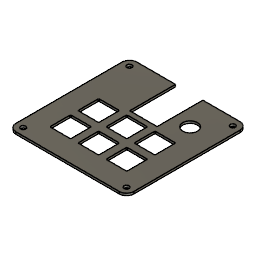
Full+Skyboard (Autodesk Fusion 360 archive; units mm, degrees)
design "TopPart"
part number: 2026-01-17-14-14-09-659
Autodesk Fusion 360 part; units mm, degrees
sketch "Sketch1" plane through (0, 0, 0) normal (0, 0, 1) x (1, 0, 0)
  line L0 (3.025, -2.525) -> (16.025, -2.525)
  line L1 (3.025, -16.525) -> (16.025, -16.525)
  line L2 (2.525, -3.025) -> (2.525, -16.025)
  line L3 (16.525, -3.025) -> (16.525, -16.025)
  arc A0 (3.025, -2.525) -> (2.525, -3.025) centre (3.025, -3.025) ccw
  arc A1 (16.525, -3.025) -> (16.025, -2.525) centre (16.025, -3.025) ccw
  arc A2 (2.525, -16.025) -> (3.025, -16.525) centre (3.025, -16.025) ccw
  arc A3 (16.025, -16.525) -> (16.525, -16.025) centre (16.025, -16.025) ccw
  line L4 (22.075, -2.525) -> (35.075, -2.525)
  line L5 (22.075, -16.525) -> (35.075, -16.525)
  line L6 (21.575, -3.025) -> (21.575, -16.025)
  line L7 (35.575, -3.025) -> (35.575, -16.025)
  arc A4 (22.075, -2.525) -> (21.575, -3.025) centre (22.075, -3.025) ccw
  arc A5 (35.575, -3.025) -> (35.075, -2.525) centre (35.075, -3.025) ccw
  arc A6 (21.575, -16.025) -> (22.075, -16.525) centre (22.075, -16.025) ccw
  arc A7 (35.075, -16.525) -> (35.575, -16.025) centre (35.075, -16.025) ccw
  line L8 (41.125, -2.525) -> (54.125, -2.525)
  line L9 (41.125, -16.525) -> (54.125, -16.525)
  line L10 (40.625, -3.025) -> (40.625, -16.025)
  line L11 (54.625, -3.025) -> (54.625, -16.025)
  arc A8 (41.125, -2.525) -> (40.625, -3.025) centre (41.125, -3.025) ccw
  arc A9 (54.625, -3.025) -> (54.125, -2.525) centre (54.125, -3.025) ccw
  arc A10 (40.625, -16.025) -> (41.125, -16.525) centre (41.125, -16.025) ccw
  arc A11 (54.125, -16.525) -> (54.625, -16.025) centre (54.125, -16.025) ccw
  line L12 (3.025, -21.575) -> (16.025, -21.575)
  line L13 (3.025, -35.575) -> (16.025, -35.575)
  line L14 (2.525, -22.075) -> (2.525, -35.075)
  line L15 (16.525, -22.075) -> (16.525, -35.075)
  arc A12 (3.025, -21.575) -> (2.525, -22.075) centre (3.025, -22.075) ccw
  arc A13 (16.525, -22.075) -> (16.025, -21.575) centre (16.025, -22.075) ccw
  arc A14 (2.525, -35.075) -> (3.025, -35.575) centre (3.025, -35.075) ccw
  arc A15 (16.025, -35.575) -> (16.525, -35.075) centre (16.025, -35.075) ccw
  line L16 (22.075, -21.575) -> (35.075, -21.575)
  line L17 (22.075, -35.575) -> (35.075, -35.575)
  line L18 (21.575, -22.075) -> (21.575, -35.075)
  line L19 (35.575, -22.075) -> (35.575, -35.075)
  arc A16 (22.075, -21.575) -> (21.575, -22.075) centre (22.075, -22.075) ccw
  arc A17 (35.575, -22.075) -> (35.075, -21.575) centre (35.075, -22.075) ccw
  arc A18 (21.575, -35.075) -> (22.075, -35.575) centre (22.075, -35.075) ccw
  arc A19 (35.075, -35.575) -> (35.575, -35.075) centre (35.075, -35.075) ccw
  line L20 (41.125, -21.575) -> (54.125, -21.575)
  line L21 (41.125, -35.575) -> (54.125, -35.575)
  line L22 (40.625, -22.075) -> (40.625, -35.075)
  line L23 (54.625, -22.075) -> (54.625, -35.075)
  arc A20 (41.125, -21.575) -> (40.625, -22.075) centre (41.125, -22.075) ccw
  arc A21 (54.625, -22.075) -> (54.125, -21.575) centre (54.125, -22.075) ccw
  arc A22 (40.625, -35.075) -> (41.125, -35.575) centre (41.125, -35.075) ccw
  arc A23 (54.125, -35.575) -> (54.625, -35.075) centre (54.125, -35.075) ccw
  line L24 (-11.052, 31.916) -> (68.948, 31.916)
  line L25 (68.948, 31.916) -> (68.948, -50.084)
  line L26 (68.948, -50.084) -> (-11.052, -50.084)
  line L27 (-11.052, -50.084) -> (-11.052, 31.916)
  line L28 (20.198, 31.916) -> (38.698, 31.916)
  line L29 (38.698, 31.916) -> (38.698, 0.916)
  line L30 (38.698, 0.916) -> (20.198, 0.916)
  line L31 (20.198, 0.916) -> (20.198, 31.916)
  circle A24 centre (-6.052, 26.916) radius 1.7
  circle A25 centre (-6.052, -45.084) radius 1.7
  circle A26 centre (63.948, -45.084) radius 1.7
  circle A27 centre (63.948, 26.916) radius 1.7
  dimension "d1" = 80
  dimension "d2" = 82
  dimension "d4" = 13.577
  dimension "d5" = 14.509
  dimension "d6" = 18.5
  dimension "d7" = 31
  dimension "d8" = 31.25
  dimension "d9" = 3.4
  dimension "d10" = 5
  dimension "d11" = 5
  dimension "d12" = 3.4
  dimension "d13" = 5
  dimension "d14" = 5
  dimension "d15" = 3.4
  dimension "d16" = 5
  dimension "d17" = 5
  dimension "d18" = 3.4
  dimension "d19" = 5
  dimension "d20" = 5
  constraint horizontal L24
  constraint vertical L25
  constraint horizontal L26
  constraint vertical L27
  constraint horizontal L28
  constraint vertical L29
  constraint horizontal L30
  constraint vertical L31
  constraint coincident L24 L28.start
  measures "d1" distance of L24.start L24.end
  measures "d2" distance of L24.start L26.end
  measures "d4" distance of L14 L27
  measures "d5" distance of L13 L26
  measures "d6" distance of L28.start L28.end
  measures "d7" distance of L28.start L30.end
  measures "d8" distance of L27 L31
  measures "d9" diameter of A24
  measures "d10" distance of L24 A24.centre
  measures "d11" distance of L27 A24.centre
  measures "d12" diameter of A25
  measures "d13" distance of L26 A25.centre
  measures "d14" distance of L27 A25.centre
  measures "d15" diameter of A26
  measures "d16" distance of L26 A26.centre
  measures "d17" distance of L25 A26.centre
  measures "d18" diameter of A27
  measures "d19" distance of L24 A27.centre
  measures "d20" distance of L25 A27.centre
extrude "Extrude1" add sketch "Sketch1" along normal blind 1.5 contours L24 L25 L26 L27 L29 L30 L31
fillet "Fillet1" radius 5 4 edges at (-11.052, -50.084, 0.75) (-11.052, 31.916, 0.75) (68.948, -50.084, 0.75) (68.948, 31.916, 0.75)
sketch "Sketch2" plane through (0, 0, 1.5) normal (0, 0, 1) x (-1, 0, 0)
  arc A0 (-68.948, -26.916) -> (-63.948, -31.916) centre (-63.948, -26.916) ccw
  line L0 (-63.948, -31.916) -> (-38.698, -31.916)
  line L1 (-38.698, -31.916) -> (-38.698, -0.916)
  line L2 (-38.698, -0.916) -> (-20.198, -0.916)
  line L3 (-20.198, -0.916) -> (-20.198, -31.916)
  line L4 (-20.198, -31.916) -> (6.052, -31.916)
  arc A1 (6.052, -31.916) -> (11.052, -26.916) centre (6.052, -26.916) ccw
  line L5 (11.052, -26.916) -> (11.052, 45.084)
  arc A2 (11.052, 45.084) -> (6.052, 50.084) centre (6.052, 45.084) ccw
  line L6 (6.052, 50.084) -> (-63.948, 50.084)
  arc A3 (-63.948, 50.084) -> (-68.948, 45.084) centre (-63.948, 45.084) ccw
  line L7 (-68.948, 45.084) -> (-68.948, -26.916)
  arc A4 (-41.125, 2.525) -> (-40.625, 3.025) centre (-41.125, 3.025) ccw
  line L8 (-41.125, 2.525) -> (-54.125, 2.525)
  arc A5 (-54.625, 3.025) -> (-54.125, 2.525) centre (-54.125, 3.025) ccw
  line L9 (-54.625, 3.025) -> (-54.625, 16.025)
  arc A6 (-54.125, 16.525) -> (-54.625, 16.025) centre (-54.125, 16.025) ccw
  line L10 (-54.125, 16.525) -> (-41.125, 16.525)
  arc A7 (-40.625, 16.025) -> (-41.125, 16.525) centre (-41.125, 16.025) ccw
  line L11 (-40.625, 16.025) -> (-40.625, 3.025)
  arc A8 (-22.075, 2.525) -> (-21.575, 3.025) centre (-22.075, 3.025) ccw
  line L12 (-22.075, 2.525) -> (-35.075, 2.525)
  arc A9 (-35.575, 3.025) -> (-35.075, 2.525) centre (-35.075, 3.025) ccw
  line L13 (-35.575, 3.025) -> (-35.575, 16.025)
  arc A10 (-35.075, 16.525) -> (-35.575, 16.025) centre (-35.075, 16.025) ccw
  line L14 (-35.075, 16.525) -> (-22.075, 16.525)
  arc A11 (-21.575, 16.025) -> (-22.075, 16.525) centre (-22.075, 16.025) ccw
  line L15 (-21.575, 16.025) -> (-21.575, 3.025)
  circle A12 centre (-63.948, 45.084) radius 1.7
  arc A13 (-3.025, 21.575) -> (-2.525, 22.075) centre (-3.025, 22.075) ccw
  line L16 (-3.025, 21.575) -> (-16.025, 21.575)
  arc A14 (-16.525, 22.075) -> (-16.025, 21.575) centre (-16.025, 22.075) ccw
  line L17 (-16.525, 22.075) -> (-16.525, 35.075)
  arc A15 (-16.025, 35.575) -> (-16.525, 35.075) centre (-16.025, 35.075) ccw
  line L18 (-16.025, 35.575) -> (-3.025, 35.575)
  arc A16 (-2.525, 35.075) -> (-3.025, 35.575) centre (-3.025, 35.075) ccw
  line L19 (-2.525, 35.075) -> (-2.525, 22.075)
  arc A17 (-3.025, 2.525) -> (-2.525, 3.025) centre (-3.025, 3.025) ccw
  line L20 (-3.025, 2.525) -> (-16.025, 2.525)
  arc A18 (-16.525, 3.025) -> (-16.025, 2.525) centre (-16.025, 3.025) ccw
  line L21 (-16.525, 3.025) -> (-16.525, 16.025)
  arc A19 (-16.025, 16.525) -> (-16.525, 16.025) centre (-16.025, 16.025) ccw
  line L22 (-16.025, 16.525) -> (-3.025, 16.525)
  arc A20 (-2.525, 16.025) -> (-3.025, 16.525) centre (-3.025, 16.025) ccw
  line L23 (-2.525, 16.025) -> (-2.525, 3.025)
  circle A21 centre (6.052, 45.084) radius 1.7
  arc A22 (-41.125, 21.575) -> (-40.625, 22.075) centre (-41.125, 22.075) ccw
  line L24 (-41.125, 21.575) -> (-54.125, 21.575)
  arc A23 (-54.625, 22.075) -> (-54.125, 21.575) centre (-54.125, 22.075) ccw
  line L25 (-54.625, 22.075) -> (-54.625, 35.075)
  arc A24 (-54.125, 35.575) -> (-54.625, 35.075) centre (-54.125, 35.075) ccw
  line L26 (-54.125, 35.575) -> (-41.125, 35.575)
  arc A25 (-40.625, 35.075) -> (-41.125, 35.575) centre (-41.125, 35.075) ccw
  line L27 (-40.625, 35.075) -> (-40.625, 22.075)
  circle A26 centre (6.052, -26.916) radius 1.7
  arc A27 (-22.075, 21.575) -> (-21.575, 22.075) centre (-22.075, 22.075) ccw
  line L28 (-22.075, 21.575) -> (-35.075, 21.575)
  arc A28 (-35.575, 22.075) -> (-35.075, 21.575) centre (-35.075, 22.075) ccw
  line L29 (-35.575, 22.075) -> (-35.575, 35.075)
  arc A29 (-35.075, 35.575) -> (-35.575, 35.075) centre (-35.075, 35.075) ccw
  line L30 (-35.075, 35.575) -> (-22.075, 35.575)
  arc A30 (-21.575, 35.075) -> (-22.075, 35.575) centre (-22.075, 35.075) ccw
  line L31 (-21.575, 35.075) -> (-21.575, 22.075)
  circle A31 centre (-63.948, -26.916) radius 1.7
  circle A32 centre (-50.098, -11.875) radius 5
  dimension "d28" = 10
  dimension "d29" = 14.4
  dimension "d30" = 11.4
  measures "d28" diameter of A32
  measures "d29" distance of L8 A32.centre
  measures "d30" distance of L1 A32.centre
extrude "Extrude2" cut sketch "Sketch2" against normal blind 5 contours A32
